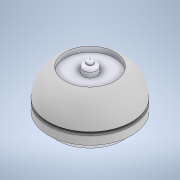
# Autodesk Inventor part: camera
Saved by Autodesk Inventor 2022.2 (Build 262287000, 287)
## iProperties
Created: 2022-02-22
Part Number: camera
Material: Generic
Document SubType Name: Modeling
Designer: ONG
Density: 1 g/cm^3
Appearance: Default
Author: ONG
Autodesk Inventor part; units mm, degrees
ref_plane "YZ Plane" through (0, 0, 0) normal (1, 0, 0) x (0, 1, 0)
ref_plane "XY Plane" through (0, 0, 0) normal (0, 0, 1) x (1, 0, 0)
sketch "Sketch1" plane through (0, 0, 0) normal (0, 1, 0) x (-1, 0, 0)
  circle A0 centre (0, 0) radius 25
  dimension "d0" = 50
  constraints: 1 centre point, 1 coincident
  measures "d0" diameter of A0
extrude "Extrusion1" add sketch "Sketch1" along normal blind 30
fillet "Fillet1" radius 18 1 edges at (25, 30, 0)
chamfer "Chamfer1" distance 5 angle 45 1 edges at (25, 0, 0)
sketch "Sketch2" plane through (0, 30, 0) normal (0, 1, 0) x (1, 0, 0)
  line L0 (0, 0) -> (6.5883, 0)
  line L1 (6.5883, 0) -> (-7, 0)
  circle A0 centre (0, 0) radius 7 projected
  circle A1 centre (0, 0) radius 6.5883
  circle A2 centre (0, 0) radius 25
  circle A3 centre (0, 0) radius 15
  dimension "d7" = 30
  constraints: 4 end point, 3 centre point, 3 coincident, 1 horizontal, 1 horizontal alignment, 1 point on line, 1 other
  measures "d7" diameter of A3
extrude "Extrusion2" cut sketch "Sketch2" against normal blind 5 contours L1 A1 L0 | L0 A1 L1 | A0 | A3
sketch "Sketch3" plane through (0, 25, 0) normal (0, 1, 0) x (1, 0, 0)
  circle A0 centre (0, 0) radius 4
  dimension "d10" = 8
  constraints: 1 centre point, 1 coincident
  measures "d10" diameter of A0
extrude "Extrusion3" add sketch "Sketch3" along normal blind 5
fillet "Fillet2" radius 2 1 edges at (-4, 30, 0)
ref_plane "Work Plane1" through (0, 12, 0) normal (0, 1, 0) x (-1, 0, 0)
sketch "Sketch4" plane through (0, 12, 0) normal (0, 1, 0) x (-1, 0, 0)
  circle A0 centre (0, 0) radius 4 projected
  circle A1 centre (0, 0) radius 25
  circle A2 centre (0, 0) radius 2 projected
  circle A3 centre (0, 0) radius 15
  dimension "d21" = 30
  constraints: 2 centre point, 2 coincident
  measures "d21" diameter of A3
sketch "Sketch5" plane through (0, 30, 0) normal (0, 1, 0) x (1, 0, 0)
  circle A0 centre (0, 0) radius 2
  circle A1 centre (0, 0) radius 1.75
  dimension "d17" = 3.5
  constraints: 2 centre point, 2 coincident
  measures "d17" diameter of A1
extrude "Extrusion5" add sketch "Sketch5" along normal blind 2 contours A1
fillet "Fillet3" radius 1.5 1 edges at (-1.75, 32, 0)
extrude "Extrusion6" cut sketch "Sketch4" against normal blind 2 contours A1
body "Solid1"
